hexlight (Autodesk Fusion 360 design; units mm, degrees)
Autodesk Fusion 360 part; units mm, degrees
note: some values were not read from the file. Chosen so that the rebuilt part matches the saved one: which face or edge a step refers to. Set by a fixed rule: which sketch regions a step uses.
sketch "Sketch1" plane through (0, 0, 0) normal (0, 0, 1) x (1, 0, 0)
  line L0 (86.6025, -50) -> (86.6025, 50)
  line L1 (86.6025, 50) -> (0, 100)
  line L2 (0, 100) -> (-86.6025, 50)
  line L3 (-86.6025, 50) -> (-86.6025, -50)
  line L4 (-86.6025, -50) -> (0, -100)
  line L5 (0, -100) -> (86.6025, -50)
  line L6 (0, -104.6188) -> (90.6025, -52.3094)
  line L7 (90.6025, -52.3094) -> (90.6025, 52.3094)
  line L8 (90.6025, 52.3094) -> (0, 104.6188)
  line L9 (0, 104.6188) -> (-90.6025, 52.3094)
  line L10 (-90.6025, 52.3094) -> (-90.6025, -52.3094)
  line L11 (-90.6025, -52.3094) -> (0, -104.6188)
  line L12 (0, 0) -> (0, -155)
  line L13 (0, -98.8453) -> (85.6025, -49.4226)
  line L14 (85.6025, -49.4226) -> (85.6025, 49.4226)
  line L15 (85.6025, 49.4226) -> (0, 98.8453)
  line L16 (0, 98.8453) -> (-85.6025, 49.4226)
  line L17 (-85.6025, 49.4226) -> (-85.6025, -49.4226)
  line L18 (-85.6025, -49.4226) -> (0, -98.8453)
  line L19 (0, -97.4597) -> (84.4025, -48.7298)
  line L20 (84.4025, -48.7298) -> (84.4025, 48.7298)
  line L21 (84.4025, 48.7298) -> (0, 97.4597)
  line L22 (0, 97.4597) -> (-84.4025, 48.7298)
  line L23 (-84.4025, 48.7298) -> (-84.4025, -48.7298)
  line L24 (-84.4025, -48.7298) -> (0, -97.4597)
  line L25 (-85.6025, -44.4226) -> (-84.4025, -44.4226)
  line L26 (-81.2724, -51.9226) -> (-80.6724, -50.8834)
  line L27 (-56.9017, -65.9931) -> (-56.3017, -64.9539)
  line L28 (-28.2008, -82.5635) -> (-27.6008, -81.5243)
  line L29 (-60.6318, -62.4539) -> (-61.2318, -63.4931)
  line L30 (-55.0893, -65.6539) -> (-55.6893, -66.6931)
  line L31 (-31.931, -79.0243) -> (-32.531, -80.0635)
  line L32 (-23.2707, -84.0243) -> (-23.8707, -85.0635)
  line L33 (61.1318, -62.1652) -> (61.7318, -63.2044)
  line L34 (52.4716, -67.1652) -> (53.0716, -68.2044)
  line L35 (29.3133, -80.5356) -> (29.9133, -81.5749)
  line L36 (23.7707, -83.7356) -> (24.3707, -84.7749)
  line L37 (4.3301, -96.3453) -> (3.7301, -95.3061)
  line L38 (-4.3301, -96.3453) -> (-3.7301, -95.3061)
  line L39 (84.4025, 21.8591) -> (85.6025, 21.8591)
  line L40 (84.4025, 11.8591) -> (85.6025, 11.8591)
  line L41 (84.4025, -14.8818) -> (85.6025, -14.8818)
  line L42 (84.4025, -21.2818) -> (85.6025, -21.2818)
  line L43 (85.6025, -44.4226) -> (84.4025, -44.4226)
  line L44 (81.2724, -51.9226) -> (80.6724, -50.8834)
  line L45 (23.2707, 84.0243) -> (23.8707, 85.0635)
  line L46 (31.931, 79.0243) -> (32.531, 80.0635)
  line L47 (55.0893, 65.6539) -> (55.6893, 66.6931)
  line L48 (60.6318, 62.4539) -> (61.2318, 63.4931)
  line L49 (81.2724, 51.9226) -> (80.6724, 50.8834)
  line L50 (85.6025, 44.4226) -> (84.4025, 44.4226)
  line L51 (-61.1318, 62.1652) -> (-61.7318, 63.2044)
  line L52 (-52.4716, 67.1652) -> (-53.0716, 68.2044)
  line L53 (-29.3133, 80.5356) -> (-29.9133, 81.5749)
  line L54 (-23.7707, 83.7356) -> (-24.3707, 84.7749)
  line L55 (-4.3301, 96.3453) -> (-3.7301, 95.3061)
  line L56 (4.3301, 96.3453) -> (3.7301, 95.3061)
  line L57 (-84.4025, -21.8591) -> (-85.6025, -21.8591)
  line L58 (-84.4025, -11.8591) -> (-85.6025, -11.8591)
  line L59 (-84.4025, 14.8818) -> (-85.6025, 14.8818)
  line L60 (-84.4025, 21.2818) -> (-85.6025, 21.2818)
  line L61 (-85.6025, 44.4226) -> (-84.4025, 44.4226)
  line L62 (-81.2724, 51.9226) -> (-80.6724, 50.8834)
  line L63 (-85.6025, -41.9226) -> (-84.4025, -41.9226)
  line L64 (-78.5073, -52.1334) -> (-79.1073, -53.1726)
  line L65 (-6.4952, -95.0953) -> (-5.8952, -94.0561)
  line L66 (5.8952, -94.0561) -> (6.4952, -95.0953)
  line L67 (79.1073, -53.1726) -> (78.5073, -52.1334)
  line L68 (84.4025, -41.9226) -> (85.6025, -41.9226)
  line L69 (85.6025, 41.9226) -> (84.4025, 41.9226)
  line L70 (78.5073, 52.1334) -> (79.1073, 53.1726)
  line L71 (6.4952, 95.0953) -> (5.8952, 94.0561)
  line L72 (-5.8952, 94.0561) -> (-6.4952, 95.0953)
  line L73 (-79.1073, 53.1726) -> (-78.5073, 52.1334)
  line L74 (-84.4025, 41.9226) -> (-85.6025, 41.9226)
  line L75 (-84.4025, -41.9226) -> (-83.1025, -41.9226)
  line L76 (-83.1025, -41.9226) -> (-83.1025, -44.4226)
  line L77 (-83.1025, -44.4226) -> (-84.4025, -44.4226)
  line L78 (-80.6724, -50.8834) -> (-80.0224, -49.7576)
  line L79 (-78.5073, -52.1334) -> (-77.8573, -51.0076)
  line L80 (-77.8573, -51.0076) -> (-80.0224, -49.7576)
  line L81 (-5.8952, -94.0561) -> (-5.2452, -92.9302)
  line L82 (-5.2452, -92.9302) -> (-3.0801, -94.1802)
  line L83 (-3.0801, -94.1802) -> (-3.7301, -95.3061)
  line L84 (3.7301, -95.3061) -> (3.0801, -94.1802)
  line L85 (5.2452, -92.9302) -> (3.0801, -94.1802)
  line L86 (5.8952, -94.0561) -> (5.2452, -92.9302)
  line L87 (78.5073, -52.1334) -> (77.8573, -51.0076)
  line L88 (77.8573, -51.0076) -> (80.0224, -49.7576)
  line L89 (80.0224, -49.7576) -> (80.6724, -50.8834)
  line L90 (84.4025, -44.4226) -> (83.1025, -44.4226)
  line L91 (83.1025, -41.9226) -> (83.1025, -44.4226)
  line L92 (84.4025, -41.9226) -> (83.1025, -41.9226)
  line L93 (84.4025, 41.9226) -> (83.1025, 41.9226)
  line L94 (83.1025, 41.9226) -> (83.1025, 44.4226)
  line L95 (83.1025, 44.4226) -> (84.4025, 44.4226)
  line L96 (80.6724, 50.8834) -> (80.0224, 49.7576)
  line L97 (77.8573, 51.0076) -> (80.0224, 49.7576)
  line L98 (78.5073, 52.1334) -> (77.8573, 51.0076)
  line L99 (5.8952, 94.0561) -> (5.2452, 92.9302)
  line L100 (5.2452, 92.9302) -> (3.0801, 94.1802)
  line L101 (3.0801, 94.1802) -> (3.7301, 95.3061)
  line L102 (-3.7301, 95.3061) -> (-3.0801, 94.1802)
  line L103 (-5.2452, 92.9302) -> (-3.0801, 94.1802)
  line L104 (-5.8952, 94.0561) -> (-5.2452, 92.9302)
  line L105 (-78.5073, 52.1334) -> (-77.8573, 51.0076)
  line L106 (-77.8573, 51.0076) -> (-80.0224, 49.7576)
  line L107 (-80.0224, 49.7576) -> (-80.6724, 50.8834)
  line L108 (-84.4025, 44.4226) -> (-83.1025, 44.4226)
  line L109 (-83.1025, 41.9226) -> (-83.1025, 44.4226)
  line L110 (-84.4025, 41.9226) -> (-83.1025, 41.9226)
  dimension "d1" = 100
  dimension "d2" = 4
  dimension "d7" = 1
  dimension "d8" = 1.2
  dimension "d9" = 5
  dimension "d10" = 5
  dimension "d11" = 98.8453
  dimension "d12" = 33.1409
  dimension "d13" = 66.2818
  dimension "d14" = 5
  dimension "d15" = 5
  dimension "d16" = 1.4
  dimension "d17" = 5
  dimension "d19" = 360
  dimension "d22" = 2.5
  dimension "d23" = 2.5
  dimension "d25" = 360
  dimension "d27" = 1.3
  dimension "d29" = 1.3
  dimension "d31" = 360
  constraint coincident L12.start origin
  constraint vertical L12
  constraint coincident L4.end L12
  constraint coincident L6.start L12
  constraint coincident L12 L13.start
  constraint coincident L12 L19.start
  constraint coincident L17 L25.start
  constraint coincident L23 L25.end
  constraint perpendicular L23 L25
  constraint coincident L18 L26.start
  constraint coincident L24 L26.end
  constraint perpendicular L24 L26
  constraint coincident L18 L27.start
  constraint coincident L24 L27.end
  constraint perpendicular L24 L27
  constraint coincident L18 L28.start
  constraint coincident L24 L28.end
  constraint perpendicular L24 L28
  constraint coincident L24 L29.start
  constraint coincident L18 L29.end
  constraint perpendicular L18 L29
  constraint coincident L24 L30.start
  constraint coincident L18 L30.end
  constraint perpendicular L18 L30
  constraint coincident L24 L31.start
  constraint coincident L18 L31.end
  constraint perpendicular L18 L31
  constraint coincident L24 L32.start
  constraint coincident L18 L32.end
  constraint perpendicular L18 L32
  constraint coincident L17 L63.start
  constraint coincident L23 L63.end
  constraint perpendicular L23 L63
  constraint coincident L24 L64.start
  constraint coincident L18 L64.end
  constraint perpendicular L18 L64
  constraint perpendicular L23 L75
  constraint perpendicular L75 L76
  constraint collinear L25 L77
  constraint perpendicular L24 L78
  constraint perpendicular L24 L79
  constraint parallel L24 L80
  measures "d1" distance of L0.start L4.end
  measures "d2" distance of L5 L6
  measures "d7" distance of L5 L13
  measures "d8" distance of L13 L19
  measures "d9" distance of L17.end L25
  measures "d10" distance of L17.end L26
  measures "d11" distance of L13.start L17.end
  measures "d12" distance of L17.end L27.start
  measures "d13" distance of L17.end L28.start
  measures "d14" distance of L28 L32
  measures "d15" distance of L28.end L31.start
  measures "d16" distance of L27.start L30.end
  measures "d17" distance of L27.start L29.end
  measures "d22" distance of L25 L63
  measures "d23" distance of L26 L64
  measures "d27" distance of L63.end L75.end
  measures "d29" distance of L26.end L78.end
extrude "Extrude1" add sketch "Sketch1" against normal blind 0.8 contours L0 L1 L2 L3 L4 L5 | L6 L7 L8 L9 L10 L11 | L12 L13 L19 L37 | L19 L20 L21 L22 L23 L24 L75 L76 L77 L78 L79 L80 L81 L82 L83 L84 L85 L86 L87 L88 L89 L90 L91 L92 L93 L94 L95 L96 L97 L98 L99 L100 L101 L102 L103 L104 L105 L106 L107 L108 L109 L110 | L12 L18 L24 L38 | L19 L84 L85 L86 | L13 L19 L37 L66 | L18 L24 L38 L65 | L24 L81 L82 L83 | L13 L19 L36 L66 | L18 L24 L32 L65 | L13 L19 L35 L36 | L18 L24 L28 L32 | L13 L19 L34 L35 | L18 L24 L28 L31 | L13 L19 L33 L34 | L18 L24 L30 L31 | L13 L19 L33 L67 | L18 L24 L27 L30 | L19 L87 L88 L89 | L13 L19 L44 L67 | L18 L24 L27 L29 | L13 L14 L19 L20 L43 L44 | L18 L24 L29 L64 | L18 L24 L26 L64 | L24 L78 L79 L80 | L20 L90 L91 L92 | L14 L20 L43 L68 | L17 L18 L23 L24 L25 L26 | L14 L20 L42 L68 | L14 L20 L41 L42 | L17 L23 L25 L63 | L23 L75 L76 L77 | L14 L20 L40 L41 | L17 L23 L57 L63 | L14 L20 L39 L40 | L17 L23 L57 L58 | L14 L20 L39 L69 | L17 L23 L58 L59 | L20 L93 L94 L95 | L14 L20 L50 L69 | L17 L23 L59 L60 | L14 L15 L20 L21 L49 L50 | L17 L23 L60 L74 | L17 L23 L61 L74 | L23 L108 L109 L110 | L21 L96 L97 L98 | L15 L21 L49 L70 | L16 L17 L22 L23 L61 L62 | L15 L21 L48 L70 | L15 L21 L47 L48 | L16 L22 L62 L73 | L22 L105 L106 L107 | L15 L21 L46 L47 | L16 L22 L51 L73 | L15 L21 L45 L46 | L16 L22 L51 L52 | L15 L21 L45 L71 | L16 L22 L52 L53 | L21 L99 L100 L101 | L15 L21 L56 L71 | L16 L22 L53 L54 | L15 L16 L21 L22 L55 L56 | L16 L22 L54 L72 | L16 L22 L55 L72 | L22 L102 L103 L104
extrude "Extrude2" add sketch "Sketch1" along normal blind 12 contours L6 L7 L8 L9 L10 L11
extrude "Extrude3" add sketch "Sketch1" along normal blind 9.5 contours L19 L84 L85 L86 | L13 L19 L37 L66 | L18 L24 L38 L65 | L24 L81 L82 L83 | L13 L19 L35 L36 | L18 L24 L28 L32 | L18 L24 L28 L31 | L13 L19 L33 L34 | L18 L24 L27 L30 | L19 L87 L88 L89 | L13 L19 L44 L67 | L18 L24 L27 L29 | L18 L24 L26 L64 | L24 L78 L79 L80 | L20 L90 L91 L92 | L14 L20 L43 L68 | L14 L20 L41 L42 | L17 L23 L25 L63 | L23 L75 L76 L77 | L14 L20 L39 L40 | L17 L23 L57 L58 | L20 L93 L94 L95 | L14 L20 L50 L69 | L17 L23 L59 L60 | L17 L23 L61 L74 | L23 L108 L109 L110 | L21 L96 L97 L98 | L15 L21 L49 L70 | L15 L21 L47 L48 | L16 L22 L62 L73 | L22 L105 L106 L107 | L15 L21 L45 L46 | L16 L22 L51 L52 | L21 L99 L100 L101 | L15 L21 L56 L71 | L16 L22 L53 L54 | L16 L22 L55 L72 | L22 L102 L103 L104
ref_plane "WorkPlane1" through (-15.8013, 27.3686, 6) normal (0.5, -0.866025, 0) x (0.866025, 0.5, 0)
sketch "Sketch4" plane through (-43.3013, 75, 0) normal (0.5, -0.866025, 0) x (0.866025, 0.5, 0)
  line L0 (-50, 0) -> (50, 0)
  line L1 (50, 0) -> (50, 12)
  line L2 (50, 12) -> (-50, 12)
  line L3 (-50, 12) -> (-50, 0)
  line L4 (10, 0) -> (6, 0)
  line L5 (6, 0) -> (6, 0.5)
  line L6 (6, 0.5) -> (10, 0.5)
  line L7 (10, 0.5) -> (10, 0)
  line L8 (6, 0.5) -> (10, 0.5)
  line L9 (10, 0.5) -> (10, 3)
  line L10 (10, 3) -> (6, 3)
  line L11 (6, 3) -> (6, 0.5)
  line L12 (10, 3) -> (6, 3)
  line L13 (6, 3) -> (6, 5.12)
  line L14 (10, 5.1981) -> (10, 3)
  line L15 (6, 5.12) -> (6, 10)
  line L16 (6, 10) -> (10, 10)
  line L17 (10, 10) -> (10, 5.1981)
  line L18 (6, 7) -> (10, 7)
  line L19 (10, 10) -> (6, 10)
  line L20 (6, 10) -> (6, 12)
  line L21 (6, 12) -> (10, 12)
  line L22 (10, 12) -> (10, 10)
  line L23 (6, 6.4) -> (-7, 6.4)
  line L24 (-7, 6.4) -> (-7, 3.6)
  line L25 (-7, 3.6) -> (6, 3.6)
  line L26 (6, 3.6) -> (6, 6.4)
  line L27 (-5, 6.4) -> (-5, 3.6)
  dimension "d33" = 0.5
  dimension "d34" = 2.5
  dimension "d35" = 10
  dimension "d36" = 3
  dimension "d37" = 4
  dimension "d38" = 40
  dimension "d86" = 0.6
  dimension "d87" = 0.6
  dimension "d129" = 2
  dimension "d130" = 11
  constraint horizontal L4
  constraint vertical L5
  constraint horizontal L6
  constraint vertical L7
  constraint coincident L0 L4.start
  constraint horizontal L8
  constraint vertical L9
  constraint horizontal L10
  constraint vertical L11
  constraint coincident L6.end L9
  constraint horizontal L12
  constraint vertical L13
  constraint vertical L14
  constraint coincident L10.end L13
  constraint vertical L15
  constraint horizontal L16
  constraint vertical L17
  constraint coincident L13 L15.start
  constraint coincident L15 L18.start
  constraint coincident L17 L18.end
  constraint perpendicular L17 L18
  constraint coincident L13.end L15.start
  constraint horizontal L19
  constraint vertical L20
  constraint horizontal L21
  constraint vertical L22
  constraint coincident L2 L20.end
  constraint coincident L15.end L20
  constraint horizontal L23
  constraint vertical L24
  constraint horizontal L25
  constraint vertical L26
  constraint coincident L15 L23.start
  constraint coincident L23 L27.start
  constraint coincident L25 L27.end
  constraint perpendicular L25 L27
  measures "d33" distance of L4 L6
  measures "d34" distance of L6.end L9.end
  measures "d35" distance of L4 L16
  measures "d36" distance of L16 L18
  measures "d37" distance of L15.end L16.end
  measures "d38" distance of L0.end L14
  measures "d86" distance of L18 L23
  measures "d87" distance of L10 L25
  measures "d129" distance of L24 L27
  measures "d130" distance of L26 L27
sketch "Sketch5" plane through (0, 0, 12) normal (0, 0, 1) x (-1, 0, 0)
  line L0 (-86.6025, 50) -> (0, 100)
  line L1 (0, 100) -> (86.6025, 50)
  line L2 (86.6025, 50) -> (86.6025, -50)
  line L3 (86.6025, -50) -> (0, -100)
  line L4 (0, -100) -> (-86.6025, -50)
  line L5 (-86.6025, -50) -> (-86.6025, 50)
  line L6 (90.6025, 52.3094) -> (0, 104.6188)
  line L7 (0, 104.6188) -> (-90.6025, 52.3094)
  line L8 (-90.6025, 52.3094) -> (-90.6025, -52.3094)
  line L9 (-90.6025, -52.3094) -> (0, -104.6188)
  line L10 (0, -104.6188) -> (90.6025, -52.3094)
  line L11 (90.6025, -52.3094) -> (90.6025, 52.3094)
  line L12 (34.641, -80) -> (42.641, -80)
  line L13 (42.641, -80) -> (46.1051, -78)
  line L14 (38.1051, -78) -> (46.1051, -78)
  line L15 (38.1051, -78) -> (34.641, -80)
  point P0 (34.641, -80)
  point P1 (38.1051, -78)
  constraint coincident P0 L12.start
  constraint coincident L10 L12.end
  constraint horizontal L12
  constraint coincident L10 L13.end
  constraint coincident P1 L14.start
  constraint parallel L12 L14
sketch "Sketch6" plane through (0, 0, 12) normal (0, 0, 1) x (1, 0, 0)
ref_plane "WorkPlane2" through (0, 0, 0) normal (0, 0, 1) x (1, 0, 0)
sketch "Sketch7" plane through (-45.3013, 78.4641, 0) normal (-0.5, 0.866025, 0) x (-0.866025, -0.5, 0)
  line L0 (-52.3094, 12) -> (-52.3094, -0.8)
  line L1 (-52.3094, -0.8) -> (52.3094, -0.8)
  line L2 (52.3094, -0.8) -> (52.3094, 12)
  line L3 (52.3094, 12) -> (-52.3094, 12)
  line L4 (-8, 10) -> (-5, 10)
  line L5 (-8, 7) -> (-5, 7)
  line L6 (-8, 3) -> (-5, 3)
  line L7 (-8, 0) -> (-5, 0)
  line L8 (5, 10) -> (7, 10)
  line L9 (7, 10) -> (7, 7)
  line L10 (7, 7) -> (5, 7)
  line L11 (5, 7) -> (5, 10)
  line L12 (7, 3) -> (5, 3)
  line L13 (5, 3) -> (5, 0)
  line L14 (5, 0) -> (7, 0)
  line L15 (7, 0) -> (7, 3)
  line L16 (5, 6.4) -> (7, 6.4)
  line L17 (7, 6.4) -> (7, 3.6)
  line L18 (7, 3.6) -> (5, 3.6)
  line L19 (5, 3.6) -> (5, 6.4)
  line L20 (-52.3094, 12) -> (52.3094, 12)
  line L21 (52.3094, 12) -> (52.3094, -0.8)
  line L22 (52.3094, -0.8) -> (-52.3094, -0.8)
  line L23 (-52.3094, -0.8) -> (-52.3094, 12)
  line L24 (0, 12) -> (-5, 12)
  line L25 (-5, 12) -> (-5, -0.8)
  line L26 (-5, -0.8) -> (0, -0.8)
  line L27 (0, -0.8) -> (0, 12)
  line L28 (0, 12) -> (5, 12)
  line L29 (5, 12) -> (5, -0.8)
  line L30 (5, -0.8) -> (0, -0.8)
  line L31 (0, -0.8) -> (0, 12)
  line L32 (-8, 12) -> (-8, -0.8)
  point P0 (0.9282, 12)
  point P1 (-3.0718, 12)
  dimension "d41" = 3
  dimension "d42" = 4
  dimension "d43" = 3
  dimension "d46" = 3
  dimension "d47" = 3
  dimension "d50" = 2
  dimension "d51" = 2
  dimension "d92" = 0.6
  dimension "d93" = 0.6
  dimension "d106" = 5
  dimension "d107" = 5
  dimension "d108" = 0.8
  dimension "d109" = 3
  constraint horizontal L8
  constraint vertical L9
  constraint horizontal L10
  constraint vertical L11
  constraint horizontal L12
  constraint vertical L13
  constraint horizontal L14
  constraint vertical L15
  constraint collinear L7 L14
  constraint collinear L5 L10
  constraint horizontal L16
  constraint vertical L17
  constraint horizontal L18
  constraint vertical L19
  constraint collinear L9 L17
  constraint collinear L11 L19
  constraint horizontal L20
  constraint vertical L21
  constraint horizontal L22
  constraint vertical L23
  constraint coincident L1.end L2.start
  constraint coincident L0.start L3.end
  constraint horizontal L24
  constraint vertical L25
  constraint horizontal L26
  constraint vertical L27
  constraint coincident L22 L25.end
  constraint midpoint L20 L24.start
  constraint horizontal L28
  constraint vertical L29
  constraint horizontal L30
  constraint vertical L31
  constraint coincident L22 L29.end
  constraint coincident L4.end L25
  constraint coincident L5.end L25
  constraint coincident L6.end L25
  constraint coincident L7.end L25
  constraint collinear L11 L29
  constraint collinear L13 L29
  constraint coincident L20 L32.start
  constraint coincident L22 L32.end
  constraint perpendicular L22 L32
  constraint coincident L4.start L32
  constraint coincident L5.start L32
  constraint coincident L6.start L32
  constraint coincident L7.start L32
  measures "d41" distance of L6 L7
  measures "d42" distance of L5 L6
  measures "d43" distance of L4 L5
  measures "d46" distance of L8.start L10.end
  measures "d47" distance of L12.end L13.end
  measures "d50" distance of L12.start L12.end
  measures "d51" distance of L8.start L8.end
  measures "d92" distance of L10 L16
  measures "d93" distance of L12 L18
  measures "d106" distance of L27 L29
  measures "d107" distance of L25 L31
  measures "d108" distance of L14 L22
  measures "d109" distance of L25 L32
sketch "Sketch15" plane through (-42.8731, 79.866, 5) normal (-0.5, 0.866025, 0) x (0.866025, 0.5, 0)
  line L0 (-7.8038, -2) -> (-9.8038, -2)
  line L1 (-9.8038, -2) -> (-9.8038, 2)
  line L2 (-9.8038, 2) -> (-7.8038, 2)
  line L3 (-7.8038, 2) -> (-7.8038, -2)
  line L4 (5.1962, -2) -> (2.1962, -2)
  line L5 (5.1962, 2) -> (2.1962, 2)
  line L6 (-7.8038, -1.4) -> (-9.8038, -1.4)
  line L7 (-9.8038, -1.4) -> (-9.8038, 1.4)
  line L8 (-9.8038, 1.4) -> (-7.8038, 1.4)
  line L9 (-7.8038, 1.4) -> (-7.8038, -1.4)
  line L10 (-7.8038, 1.4) -> (-7.8038, -1.4)
  dimension "d84" = 0.6
  dimension "d85" = 0.6
  dimension "d110" = 2
  constraint horizontal L0
  constraint vertical L1
  constraint horizontal L2
  constraint vertical L3
  constraint collinear L0 L4
  constraint collinear L2 L5
  constraint horizontal L6
  constraint vertical L7
  constraint horizontal L8
  constraint vertical L9
  constraint coincident L1 L7.end
  constraint coincident L3 L6.start
  constraint coincident L0.start L3.end
  constraint collinear L9 L10
  measures "d84" distance of L0 L6
  measures "d85" distance of L2 L8
  measures "d110" distance of L0.end L0.start
loft "Loft5" cut profiles "Sketch4", "Sketch15" section 1 contours L23 L24 L25 L27 section 2 contours L1 L3 L6 L7 L8 L9 L10
loft "Loft1" cut profiles "Sketch4", "Sketch7" section 1 contours L15 L16 L17 L18 L19 section 2 contours L4 L5 L25 L32
loft "Loft2" cut profiles "Sketch4", "Sketch7" section 1 contours L0 L4 L5 L6 L7 L8 | L6 L8 L9 L10 L11 L12 section 2 contours L6 L7 L25 L32
pattern_circular "C-Pattern1" count 6 over 360 about axis through (0, 0, 1.75) along (0, 0, 1) of 7 faces at (-35.885, 80.8214, 9) (-36.9229, 79.4524, 10) (-40.0158, 79.9761, 1) (-37.1291, 81.6427, 2) (-36.9229, 79.4524, 7) (-39.0605, 78.988, 9) (-36.9229, 79.4524, 3)
ref_plane "WorkPlane3" through (-51.0395, 68.6848, 4.75) normal (-0.866025, -0.5, 0) x (0.5, -0.866025, 0)
sketch "Sketch10" plane through (-51.0895, 68.7714, 4.75) normal (-0.866025, -0.5, 0) x (0.5, -0.866025, 0)
  line L0 (-5.5, 5.25) -> (-4.5, 5.25)
  line L1 (-4.5, 5.25) -> (-4.5, 2.25)
  line L2 (-4.5, 2.25) -> (-5.5, 2.25)
  line L3 (-5.5, 2.25) -> (-5.5, 5.25)
  line L4 (-5.5, -1.75) -> (-4.5, -1.75)
  line L5 (-4.5, -1.75) -> (-4.5, -4.75)
  line L6 (-4.5, -4.75) -> (-5.5, -4.75)
  line L7 (-5.5, -4.75) -> (-5.5, -1.75)
  line L8 (-4.5, 1.65) -> (-5.5, 1.65)
  line L9 (-5.5, 1.65) -> (-5.5, -1.15)
  line L10 (-5.5, -1.15) -> (-4.5, -1.15)
  line L11 (-4.5, -1.15) -> (-4.5, 1.65)
  line L12 (-5.5, -5.55) -> (-5.5, 7.2767)
  point P0 (-5.5, -5.55)
  dimension "d59" = 3
  dimension "d60" = 3
  dimension "d61" = 0.8
  dimension "d62" = 4
  dimension "d63" = 1
  dimension "d64" = 1
  dimension "d90" = 0.6
  dimension "d91" = 0.6
  constraint horizontal L0
  constraint vertical L1
  constraint horizontal L2
  constraint vertical L3
  constraint horizontal L4
  constraint vertical L5
  constraint horizontal L6
  constraint vertical L7
  constraint collinear L1 L5
  constraint horizontal L8
  constraint vertical L9
  constraint horizontal L10
  constraint vertical L11
  constraint collinear L5 L11
  constraint collinear L7 L9
  constraint coincident P0 L12.start
  constraint vertical L12
  constraint collinear L7 L12
  measures "d59" distance of L4.start L6.end
  measures "d60" distance of L0.start L2.end
  measures "d61" distance of L6 P0
  measures "d62" distance of L2 L4
  measures "d63" distance of L4.start L4.end
  measures "d64" distance of L1.end L2.end
  measures "d90" distance of L4 L10
  measures "d91" distance of L2 L8
loft "Loft6" [suppressed]
pattern_circular "C-Pattern5" [suppressed]
loft "Loft3" cut profiles "Sketch10", "Sketch7" section 1 contours L0 L1 L2 L3 L12 section 2 contours L8 L9 L10 L11 L29
loft "Loft4" cut profiles "Sketch10", "Sketch7" section 1 contours L4 L5 L6 L7 L12 section 2 contours L12 L13 L14 L15 L29
sketch "Sketch11" plane through (0, 0, 0) normal (0, 0, 1) x (-1, 0, 0)
  line L0 (0, -100) -> (34.641, -80)
  line L1 (38.3731, -82.4641) -> (40.9711, -80.9641)
  line L2 (86.6025, -50) -> (86.6025, -10)
  line L3 (86.6025, 50) -> (51.9615, 70)
  line L4 (0, 100) -> (-34.641, 80)
  line L5 (-86.6025, 50) -> (-86.6025, 10)
  line L6 (-48.4974, -72) -> (0, -100)
  line L7 (84.4025, -21.2818) -> (84.4025, -14.8818)
  line L8 (84.4025, -14.8818) -> (85.6025, -14.8818)
  line L9 (85.6025, -14.8818) -> (85.6025, -21.2818)
  line L10 (85.6025, -21.2818) -> (84.4025, -21.2818)
  line L11 (-4.3301, 96.3453) -> (-3.0801, 94.1802)
  line L12 (-3.0801, 94.1802) -> (-5.2452, 92.9302)
  line L13 (-5.2452, 92.9302) -> (-6.4952, 95.0953)
  line L14 (-6.4952, 95.0953) -> (-4.3301, 96.3453)
  line L15 (-84.4025, -21.8591) -> (-85.6025, -21.8591)
  line L16 (-85.6025, -21.8591) -> (-85.6025, -11.8591)
  line L17 (-85.6025, -11.8591) -> (-84.4025, -11.8591)
  line L18 (-84.4025, -11.8591) -> (-84.4025, -21.8591)
  line L19 (-23.2707, -84.0243) -> (-23.8707, -85.0635)
  line L20 (-23.8707, -85.0635) -> (-32.531, -80.0635)
  line L21 (-32.531, -80.0635) -> (-31.931, -79.0243)
  line L22 (-31.931, -79.0243) -> (-23.2707, -84.0243)
  line L23 (61.1318, -62.1652) -> (61.7318, -63.2044)
  line L24 (61.7318, -63.2044) -> (53.0716, -68.2044)
  line L25 (53.0716, -68.2044) -> (52.4716, -67.1652)
  line L26 (52.4716, -67.1652) -> (61.1318, -62.1652)
  line L27 (84.4025, 21.8591) -> (85.6025, 21.8591)
  line L28 (85.6025, 21.8591) -> (85.6025, 11.8591)
  line L29 (85.6025, 11.8591) -> (84.4025, 11.8591)
  line L30 (84.4025, 11.8591) -> (84.4025, 21.8591)
  line L31 (31.931, 79.0243) -> (23.2707, 84.0243)
  line L32 (23.2707, 84.0243) -> (23.8707, 85.0635)
  line L33 (23.8707, 85.0635) -> (32.531, 80.0635)
  line L34 (32.531, 80.0635) -> (31.931, 79.0243)
  line L35 (6.4952, 95.0953) -> (5.2452, 92.9302)
  line L36 (5.2452, 92.9302) -> (3.0801, 94.1802)
  line L37 (3.0801, 94.1802) -> (4.3301, 96.3453)
  line L38 (4.3301, 96.3453) -> (6.4952, 95.0953)
  line L39 (85.6025, 41.9226) -> (83.1025, 41.9226)
  line L40 (83.1025, 41.9226) -> (83.1025, 44.4226)
  line L41 (83.1025, 44.4226) -> (85.6025, 44.4226)
  line L42 (85.6025, 44.4226) -> (85.6025, 41.9226)
  line L43 (79.1073, -53.1726) -> (77.8573, -51.0076)
  line L44 (77.8573, -51.0076) -> (80.0224, -49.7576)
  line L45 (80.0224, -49.7576) -> (81.2724, -51.9226)
  line L46 (81.2724, -51.9226) -> (79.1073, -53.1726)
  line L47 (-6.4952, -95.0953) -> (-5.2452, -92.9302)
  line L48 (-5.2452, -92.9302) -> (-3.0801, -94.1802)
  line L49 (-3.0801, -94.1802) -> (-4.3301, -96.3453)
  line L50 (-4.3301, -96.3453) -> (-6.4952, -95.0953)
  line L51 (-85.6025, -41.9226) -> (-83.1025, -41.9226)
  line L52 (-83.1025, -41.9226) -> (-83.1025, -44.4226)
  line L53 (-83.1025, -44.4226) -> (-85.6025, -44.4226)
  line L54 (-85.6025, -44.4226) -> (-85.6025, -41.9226)
  line L55 (-61.1318, 62.1652) -> (-61.7318, 63.2044)
  line L56 (-61.7318, 63.2044) -> (-53.0716, 68.2044)
  line L57 (-53.0716, 68.2044) -> (-52.4716, 67.1652)
  line L58 (-52.4716, 67.1652) -> (-61.1318, 62.1652)
  line L59 (29.3133, -80.5356) -> (29.9133, -81.5749)
  line L60 (29.9133, -81.5749) -> (24.3707, -84.7749)
  line L61 (24.3707, -84.7749) -> (23.7707, -83.7356)
  line L62 (23.7707, -83.7356) -> (29.3133, -80.5356)
  line L63 (79.1073, 53.1726) -> (81.2724, 51.9226)
  line L64 (81.2724, 51.9226) -> (80.0224, 49.7576)
  line L65 (80.0224, 49.7576) -> (77.8573, 51.0076)
  line L66 (77.8573, 51.0076) -> (79.1073, 53.1726)
  line L67 (85.6025, -44.4226) -> (83.1025, -44.4226)
  line L68 (83.1025, -44.4226) -> (83.1025, -41.9226)
  line L69 (83.1025, -41.9226) -> (85.6025, -41.9226)
  line L70 (85.6025, -41.9226) -> (85.6025, -44.4226)
  line L71 (4.3301, -96.3453) -> (3.0801, -94.1802)
  line L72 (3.0801, -94.1802) -> (5.2452, -92.9302)
  line L73 (5.2452, -92.9302) -> (6.4952, -95.0953)
  line L74 (6.4952, -95.0953) -> (4.3301, -96.3453)
  line L75 (-81.2724, -51.9226) -> (-80.0224, -49.7576)
  line L76 (-80.0224, -49.7576) -> (-77.8573, -51.0076)
  line L77 (-77.8573, -51.0076) -> (-79.1073, -53.1726)
  line L78 (-79.1073, -53.1726) -> (-81.2724, -51.9226)
  line L79 (-85.6025, 44.4226) -> (-83.1025, 44.4226)
  line L80 (-83.1025, 44.4226) -> (-83.1025, 41.9226)
  line L81 (-83.1025, 41.9226) -> (-85.6025, 41.9226)
  line L82 (-85.6025, 41.9226) -> (-85.6025, 44.4226)
  line L83 (-79.1073, 53.1726) -> (-77.8573, 51.0076)
  line L84 (-77.8573, 51.0076) -> (-80.0224, 49.7576)
  line L85 (-80.0224, 49.7576) -> (-81.2724, 51.9226)
  line L86 (-81.2724, 51.9226) -> (-79.1073, 53.1726)
  line L87 (55.6893, 66.6931) -> (61.2318, 63.4931)
  line L88 (61.2318, 63.4931) -> (60.6318, 62.4539)
  line L89 (60.6318, 62.4539) -> (55.0893, 65.6539)
  line L90 (55.0893, 65.6539) -> (55.6893, 66.6931)
  line L91 (-29.9133, 81.5749) -> (-24.3707, 84.7749)
  line L92 (-24.3707, 84.7749) -> (-23.7707, 83.7356)
  line L93 (-23.7707, 83.7356) -> (-29.3133, 80.5356)
  line L94 (-29.3133, 80.5356) -> (-29.9133, 81.5749)
  line L95 (-85.6025, 14.8818) -> (-85.6025, 21.2818)
  line L96 (-85.6025, 21.2818) -> (-84.4025, 21.2818)
  line L97 (-84.4025, 21.2818) -> (-84.4025, 14.8818)
  line L98 (-84.4025, 14.8818) -> (-85.6025, 14.8818)
  line L99 (-55.6893, -66.6931) -> (-61.2318, -63.4931)
  line L100 (-61.2318, -63.4931) -> (-60.6318, -62.4539)
  line L101 (-60.6318, -62.4539) -> (-55.0893, -65.6539)
  line L102 (-55.0893, -65.6539) -> (-55.6893, -66.6931)
  line L103 (86.6025, 7) -> (-0.415, 7)
  line L104 (-0.415, 7) -> (-0.415, 5)
  line L105 (-0.415, 5) -> (86.6025, 5)
  line L106 (86.6025, 5) -> (86.6025, 7)
  line L107 (34.641, -80) -> (38.3731, -82.4641)
  line L108 (40.9711, -80.9641) -> (38.1051, -78)
  line L109 (38.1051, -78) -> (86.6025, -50)
  line L110 (-51.9615, -70) -> (-52.2295, -74.4641)
  line L111 (-52.2295, -74.4641) -> (-49.6314, -75.9641)
  line L112 (-49.6314, -75.9641) -> (-48.4974, -72)
  line L113 (86.6025, -10) -> (90.6025, -8)
  line L114 (90.6025, -8) -> (90.6025, -5)
  line L115 (90.6025, -5) -> (86.6025, -6)
  line L116 (86.6025, -6) -> (86.6025, 50)
  line L117 (51.9615, 70) -> (52.2295, 74.4641)
  line L118 (52.2295, 74.4641) -> (49.6314, 75.9641)
  line L119 (49.6314, 75.9641) -> (48.4974, 72)
  line L120 (48.4974, 72) -> (0, 100)
  line L121 (-34.641, 80) -> (-38.3731, 82.4641)
  line L122 (-38.3731, 82.4641) -> (-40.9711, 80.9641)
  line L123 (-40.9711, 80.9641) -> (-38.1051, 78)
  line L124 (-38.1051, 78) -> (-86.6025, 50)
  line L125 (-86.6025, 10) -> (-90.6025, 8)
  line L126 (-90.6025, 8) -> (-90.6025, 5)
  line L127 (-90.6025, 5) -> (-86.6025, 6)
  line L128 (-86.6025, 6) -> (-86.6025, -50)
  line L129 (-86.6025, -50) -> (-51.9615, -70)
  dimension "d66" = 2
  constraint horizontal L103
  constraint vertical L104
  constraint horizontal L105
  constraint vertical L106
  constraint coincident L103.end L104.start
  measures "d66" distance of L103.start L105.end
extrude "Extrude4" cut sketch "Sketch11" against normal blind 0.4 contours L103 L104 L105 L106 L116
pattern_circular "C-Pattern2" count 6 over 360 about axis through (0, 0, 1.75) along (0, 0, 1) of "Extrude4"
pattern_circular "C-Pattern3" count 6 over 360 about axis through (0, 0, 1.75) along (0, 0, 1) of 8 faces at (-53.0742, 73.4953, 10) (-53.0742, 73.4953, 3) (-53.0742, 73.4953, 7) (-53.5062, 72.9572, 9) (-52.1035, 73.767, 9) (-53.0742, 73.4953, 0) (-53.6728, 73.2459, 1) (-50.8674, 74.8656, 1)
sketch "Sketch12" plane through (0, 0, 0) normal (0, 0, 1) x (-1, 0, 0)
  line L0 (0.415, -7) -> (-86.6025, -7)
  circle A0 centre (0, 0) radius 7.5
  line L1 (49.3634, -71.5) -> (86.6025, -50)
  line L2 (86.6025, -50) -> (86.6025, -10)
  line L3 (86.6025, 50) -> (51.9615, 70)
  line L4 (0, 100) -> (-34.641, 80)
  line L5 (-86.6025, 50) -> (-86.6025, 10)
  line L6 (-86.6025, -50) -> (-51.9615, -70)
  line L7 (38.3731, -82.4641) -> (40.9711, -80.9641)
  line L8 (-55.6893, -66.6931) -> (-61.2318, -63.4931)
  line L9 (-61.2318, -63.4931) -> (-60.6318, -62.4539)
  line L10 (-60.6318, -62.4539) -> (-55.0893, -65.6539)
  line L11 (-55.0893, -65.6539) -> (-55.6893, -66.6931)
  line L12 (-29.9133, 81.5749) -> (-24.3707, 84.7749)
  line L13 (-24.3707, 84.7749) -> (-23.7707, 83.7356)
  line L14 (-23.7707, 83.7356) -> (-29.3133, 80.5356)
  line L15 (-29.3133, 80.5356) -> (-29.9133, 81.5749)
  line L16 (-4.3301, 96.3453) -> (-3.0801, 94.1802)
  line L17 (-3.0801, 94.1802) -> (-5.2452, 92.9302)
  line L18 (-5.2452, 92.9302) -> (-6.4952, 95.0953)
  line L19 (-6.4952, 95.0953) -> (-4.3301, 96.3453)
  line L20 (-84.4025, -21.8591) -> (-85.6025, -21.8591)
  line L21 (-85.6025, -21.8591) -> (-85.6025, -11.8591)
  line L22 (-85.6025, -11.8591) -> (-84.4025, -11.8591)
  line L23 (-84.4025, -11.8591) -> (-84.4025, -21.8591)
  line L24 (-23.2707, -84.0243) -> (-23.8707, -85.0635)
  line L25 (-23.8707, -85.0635) -> (-32.531, -80.0635)
  line L26 (-32.531, -80.0635) -> (-31.931, -79.0243)
  line L27 (-31.931, -79.0243) -> (-23.2707, -84.0243)
  line L28 (61.1318, -62.1652) -> (61.7318, -63.2044)
  line L29 (61.7318, -63.2044) -> (53.0716, -68.2044)
  line L30 (53.0716, -68.2044) -> (52.4716, -67.1652)
  line L31 (52.4716, -67.1652) -> (61.1318, -62.1652)
  line L32 (84.4025, 21.8591) -> (85.6025, 21.8591)
  line L33 (85.6025, 21.8591) -> (85.6025, 11.8591)
  line L34 (85.6025, 11.8591) -> (84.4025, 11.8591)
  line L35 (84.4025, 11.8591) -> (84.4025, 21.8591)
  line L36 (31.931, 79.0243) -> (23.2707, 84.0243)
  line L37 (23.2707, 84.0243) -> (23.8707, 85.0635)
  line L38 (23.8707, 85.0635) -> (32.531, 80.0635)
  line L39 (32.531, 80.0635) -> (31.931, 79.0243)
  line L40 (6.4952, 95.0953) -> (5.2452, 92.9302)
  line L41 (5.2452, 92.9302) -> (3.0801, 94.1802)
  line L42 (3.0801, 94.1802) -> (4.3301, 96.3453)
  line L43 (4.3301, 96.3453) -> (6.4952, 95.0953)
  line L44 (85.6025, 41.9226) -> (83.1025, 41.9226)
  line L45 (83.1025, 41.9226) -> (83.1025, 44.4226)
  line L46 (83.1025, 44.4226) -> (85.6025, 44.4226)
  line L47 (85.6025, 44.4226) -> (85.6025, 41.9226)
  line L48 (79.1073, -53.1726) -> (77.8573, -51.0076)
  line L49 (77.8573, -51.0076) -> (80.0224, -49.7576)
  line L50 (80.0224, -49.7576) -> (81.2724, -51.9226)
  line L51 (81.2724, -51.9226) -> (79.1073, -53.1726)
  line L52 (-6.4952, -95.0953) -> (-5.2452, -92.9302)
  line L53 (-5.2452, -92.9302) -> (-3.0801, -94.1802)
  line L54 (-3.0801, -94.1802) -> (-4.3301, -96.3453)
  line L55 (-4.3301, -96.3453) -> (-6.4952, -95.0953)
  line L56 (-85.6025, -41.9226) -> (-83.1025, -41.9226)
  line L57 (-83.1025, -41.9226) -> (-83.1025, -44.4226)
  line L58 (-83.1025, -44.4226) -> (-85.6025, -44.4226)
  line L59 (-85.6025, -44.4226) -> (-85.6025, -41.9226)
  line L60 (-61.1318, 62.1652) -> (-61.7318, 63.2044)
  line L61 (-61.7318, 63.2044) -> (-53.0716, 68.2044)
  line L62 (-53.0716, 68.2044) -> (-52.4716, 67.1652)
  line L63 (-52.4716, 67.1652) -> (-61.1318, 62.1652)
  line L64 (29.3133, -80.5356) -> (29.9133, -81.5749)
  line L65 (29.9133, -81.5749) -> (24.3707, -84.7749)
  line L66 (24.3707, -84.7749) -> (23.7707, -83.7356)
  line L67 (23.7707, -83.7356) -> (29.3133, -80.5356)
  line L68 (79.1073, 53.1726) -> (81.2724, 51.9226)
  line L69 (81.2724, 51.9226) -> (80.0224, 49.7576)
  line L70 (80.0224, 49.7576) -> (77.8573, 51.0076)
  line L71 (77.8573, 51.0076) -> (79.1073, 53.1726)
  line L72 (85.6025, -44.4226) -> (83.1025, -44.4226)
  line L73 (83.1025, -44.4226) -> (83.1025, -41.9226)
  line L74 (83.1025, -41.9226) -> (85.6025, -41.9226)
  line L75 (85.6025, -41.9226) -> (85.6025, -44.4226)
  line L76 (4.3301, -96.3453) -> (3.0801, -94.1802)
  line L77 (3.0801, -94.1802) -> (5.2452, -92.9302)
  line L78 (5.2452, -92.9302) -> (6.4952, -95.0953)
  line L79 (6.4952, -95.0953) -> (4.3301, -96.3453)
  line L80 (-81.2724, -51.9226) -> (-80.0224, -49.7576)
  line L81 (-80.0224, -49.7576) -> (-77.8573, -51.0076)
  line L82 (-77.8573, -51.0076) -> (-79.1073, -53.1726)
  line L83 (-79.1073, -53.1726) -> (-81.2724, -51.9226)
  line L84 (-85.6025, 44.4226) -> (-83.1025, 44.4226)
  line L85 (-83.1025, 44.4226) -> (-83.1025, 41.9226)
  line L86 (-83.1025, 41.9226) -> (-85.6025, 41.9226)
  line L87 (-85.6025, 41.9226) -> (-85.6025, 44.4226)
  line L88 (-79.1073, 53.1726) -> (-77.8573, 51.0076)
  line L89 (-77.8573, 51.0076) -> (-80.0224, 49.7576)
  line L90 (-80.0224, 49.7576) -> (-81.2724, 51.9226)
  line L91 (-81.2724, 51.9226) -> (-79.1073, 53.1726)
  line L92 (85.6025, -14.8818) -> (85.6025, -21.2818)
  line L93 (85.6025, -21.2818) -> (84.4025, -21.2818)
  line L94 (84.4025, -21.2818) -> (84.4025, -14.8818)
  line L95 (84.4025, -14.8818) -> (85.6025, -14.8818)
  line L96 (55.6893, 66.6931) -> (61.2318, 63.4931)
  line L97 (61.2318, 63.4931) -> (60.6318, 62.4539)
  line L98 (60.6318, 62.4539) -> (55.0893, 65.6539)
  line L99 (55.0893, 65.6539) -> (55.6893, 66.6931)
  line L100 (-85.6025, 14.8818) -> (-85.6025, 21.2818)
  line L101 (-85.6025, 21.2818) -> (-84.4025, 21.2818)
  line L102 (-84.4025, 21.2818) -> (-84.4025, 14.8818)
  line L103 (-84.4025, 14.8818) -> (-85.6025, 14.8818)
  line L104 (34.641, -80) -> (38.3731, -82.4641)
  line L105 (40.9711, -80.9641) -> (38.1051, -78)
  line L106 (86.6025, -10) -> (90.6025, -8)
  line L107 (90.6025, -8) -> (90.6025, -5)
  line L108 (90.6025, -5) -> (86.6025, -6)
  line L109 (86.6025, -6) -> (86.6025, 5)
  line L110 (86.6025, 7) -> (86.6025, 50)
  line L111 (51.9615, 70) -> (52.2295, 74.4641)
  line L112 (52.2295, 74.4641) -> (49.6314, 75.9641)
  line L113 (49.6314, 75.9641) -> (48.4974, 72)
  line L114 (48.4974, 72) -> (38.9711, 77.5)
  line L115 (37.2391, 78.5) -> (0, 100)
  line L116 (-34.641, 80) -> (-38.3731, 82.4641)
  line L117 (-38.3731, 82.4641) -> (-40.9711, 80.9641)
  line L118 (-40.9711, 80.9641) -> (-38.1051, 78)
  line L119 (-38.1051, 78) -> (-47.6314, 72.5)
  line L120 (-49.3634, 71.5) -> (-86.6025, 50)
  line L121 (-86.6025, 10) -> (-90.6025, 8)
  line L122 (-90.6025, 8) -> (-90.6025, 5)
  line L123 (-90.6025, 5) -> (-86.6025, 6)
  line L124 (-86.6025, 6) -> (-86.6025, -5)
  line L125 (-86.6025, -7) -> (-86.6025, -50)
  line L126 (-51.9615, -70) -> (-52.2295, -74.4641)
  line L127 (-52.2295, -74.4641) -> (-49.6314, -75.9641)
  line L128 (-49.6314, -75.9641) -> (-48.4974, -72)
  line L129 (-48.4974, -72) -> (-38.9711, -77.5)
  line L130 (-37.2391, -78.5) -> (0, -100)
  line L131 (0, -100) -> (34.641, -80)
  line L132 (38.1051, -78) -> (47.6314, -72.5)
  dimension "d132" = 15
  constraint coincident A0.centre origin
  measures "d132" diameter of A0
sketch "Sketch16" plane through (-43.3013, 75, 0) normal (0.5, -0.866025, 0) x (0.866025, 0.5, 0)
  line L0 (-7, 0) -> (-7, -0.4)
  line L1 (-5, -0.4) -> (-5, 0)
  line L2 (-5, 0) -> (6, 0)
  line L3 (6, 3) -> (10, 3)
  line L4 (50, 0) -> (50, 12)
  line L5 (50, 12) -> (-50, 12)
  line L6 (-50, 12) -> (-50, 0)
  line L7 (10, 7) -> (6, 7)
  line L8 (6, 10) -> (10, 10)
  line L9 (-7, -0.4) -> (-5, -0.4)
  line L10 (-7, 6.4) -> (-5, 6.4)
  line L11 (-5, 6.4) -> (-5, 3.6)
  line L12 (-5, 3.6) -> (-7, 3.6)
  line L13 (6, 0) -> (6, 3)
  line L14 (10, 3) -> (10, 0)
  line L15 (6, 7) -> (6, 10)
  line L16 (10, 10) -> (10, 7)
  line L17 (-7, 3.6) -> (-7, 6.4)
  line L18 (10, 0) -> (50, 0)
  line L19 (-50, 0) -> (-7, 0)
extrude "Extrude5" cut sketch "Sketch12" against normal blind 0.4 contours A0
sketch "Sketch13" plane through (43.3013, 75, 0) normal (-0.5, -0.866025, 0) x (0.866025, -0.5, 0)
  line L0 (-7, 0) -> (-7, -0.4)
  line L1 (-7, -0.4) -> (-5, -0.4)
  line L2 (-5, -0.4) -> (-5, 0)
  line L3 (-5, 0) -> (6, 0)
  line L4 (50, 0) -> (50, 12)
  line L5 (50, 12) -> (-50, 12)
  line L6 (-50, 12) -> (-50, 0)
  line L7 (-5, -0.4) -> (-7, -0.4)
  line L8 (-7, -0.4) -> (-7, 6.4)
  line L9 (-7, 6.4) -> (-5, 6.4)
  line L10 (-5, 6.4) -> (-5, -0.4)
  line L11 (6, 0) -> (6, 3)
  line L12 (6, 3) -> (10, 3)
  line L13 (10, 3) -> (10, 0)
  line L14 (10, 0) -> (50, 0)
  line L15 (-50, 0) -> (-7, 0)
  line L16 (10, 7) -> (6, 7)
  line L17 (6, 7) -> (6, 10)
  line L18 (6, 10) -> (10, 10)
  line L19 (10, 10) -> (10, 7)
  constraint horizontal L7
  constraint vertical L8
  constraint horizontal L9
  constraint vertical L10
  constraint coincident L1.end L2.start
  constraint coincident L0.end L1.start
extrude "Extrude6" cut sketch "Sketch13" against normal blind 0.5 contours L0 L1 L2 L7 L8 L9 L10
pattern_circular "C-Pattern4" count 6 over 360 about axis through (0, 0, 1.75) along (0, 0, 1) of "Extrude6"
sketch "Sketch18" plane through (0, 0, 12) normal (0, 0, 1) x (-1, 0, 0)
  line L0 (-86.6025, 50) -> (0, 100)
  line L1 (0, 100) -> (86.6025, 50)
  line L2 (86.6025, 50) -> (86.6025, -50)
  line L3 (86.6025, -50) -> (0, -100)
  line L4 (0, -100) -> (-86.6025, -50)
  line L5 (-86.6025, -50) -> (-86.6025, 50)
  line L6 (90.6025, 52.3094) -> (0, 104.6188)
  line L7 (0, 104.6188) -> (-90.6025, 52.3094)
  line L8 (-90.6025, 52.3094) -> (-90.6025, -52.3094)
  line L9 (-90.6025, -52.3094) -> (0, -104.6188)
  line L10 (0, -104.6188) -> (90.6025, -52.3094)
  line L11 (90.6025, -52.3094) -> (90.6025, 52.3094)
  line L12 (86.6025, -50) -> (-86.6025, 50)
  constraint coincident L2.end L3.start
  constraint coincident L0.start L5.end
ref_plane "WorkPlane4" through (0, 0, 12) normal (0.5, 0.866025, 0) x (0.866025, -0.5, 0)
sketch "Sketch21" plane through (0, 0, 12) normal (0, 0, 1) x (-1, 0, 0)
  line L0 (-86.6025, 50) -> (0, 100)
  line L1 (0, 100) -> (86.6025, 50)
  line L2 (86.6025, 50) -> (86.6025, -50)
  line L3 (86.6025, -50) -> (0, -100)
  line L4 (0, -100) -> (-86.6025, -50)
  line L5 (-86.6025, -50) -> (-86.6025, 50)
  line L6 (90.6025, 52.3094) -> (0, 104.6188)
  line L7 (0, 104.6188) -> (-90.6025, 52.3094)
  line L8 (-90.6025, 52.3094) -> (-90.6025, -52.3094)
  line L9 (-90.6025, -52.3094) -> (0, -104.6188)
  line L10 (0, -104.6188) -> (90.6025, -52.3094)
  line L11 (90.6025, -52.3094) -> (90.6025, 52.3094)
  line L12 (-86.6025, 44.5) -> (-88.8025, 44.5)
  line L13 (-88.8025, 44.5) -> (-88.8025, 32.5)
  line L14 (-88.8025, 32.5) -> (-86.6025, 32.5)
  line L15 (-86.6025, 32.5) -> (-86.6025, 44.5)
  line L16 (0, 0) -> (-110, 0)
  line L17 (-88.8025, -44.5) -> (-88.8025, -32.5)
  line L18 (-88.8025, -32.5) -> (-86.6025, -32.5)
  line L19 (-86.6025, -44.5) -> (-88.8025, -44.5)
  line L20 (-86.6025, -32.5) -> (-86.6025, -44.5)
  dimension "d112" = 2.2
  dimension "d113" = 12
  dimension "d114" = 5.5
  dimension "d119" = 110
  constraint horizontal L12
  constraint vertical L13
  constraint horizontal L14
  constraint vertical L15
  constraint coincident L5 L12.start
  constraint coincident L16.start origin
  constraint horizontal L16
  constraint symmetric L12.start L16 L19.start
  constraint symmetric L12.end L16 L17.start
  constraint symmetric L13.end L16 L17.end
  constraint symmetric L14.end L16 L18.end
  measures "d112" distance of L13.end L14.end
  measures "d113" distance of L12.end L13.end
  measures "d114" distance of L0.start L12
  measures "d119" distance of L16.start L16.end
extrude "Extrude8" cut sketch "Sketch21" against normal up to surface (12 mm away) contours L5 L12 L13 L14 L15 | L5 L17 L18 L19 L20
pattern_circular "C-Pattern6" count 6 over 360 about axis through (0, 0, 1.75) along (0, 0, 1) of "Extrude8"
sketch "Sketch22" plane through (0, 0, 0) normal (0, 0, 1) x (-1, 0, 0)
  line L0 (4.3301, -96.3453) -> (3.0801, -94.1802)
  line L1 (3.0801, -94.1802) -> (5.2452, -92.9302)
  line L2 (5.2452, -92.9302) -> (6.4952, -95.0953)
  line L3 (6.4952, -95.0953) -> (4.3301, -96.3453)
  line L4 (29.3133, -80.5356) -> (29.9133, -81.5749)
  line L5 (29.9133, -81.5749) -> (24.3707, -84.7749)
  line L6 (24.3707, -84.7749) -> (23.7707, -83.7356)
  line L7 (23.7707, -83.7356) -> (29.3133, -80.5356)
  line L8 (-23.2707, -84.0243) -> (-23.8707, -85.0635)
  line L9 (-23.8707, -85.0635) -> (-32.531, -80.0635)
  line L10 (-32.531, -80.0635) -> (-31.931, -79.0243)
  line L11 (-31.931, -79.0243) -> (-23.2707, -84.0243)
  line L12 (-15.1554, -91.25) -> (-16.2554, -93.1553)
  line L13 (-16.2554, -93.1553) -> (-5.8631, -99.1553)
  line L14 (-5.8631, -99.1553) -> (-4.7631, -97.25)
  line L15 (-4.7631, -97.25) -> (0, -100)
  line L16 (0, -100) -> (4.7631, -97.25)
  line L17 (4.7631, -97.25) -> (5.8631, -99.1553)
  line L18 (5.8631, -99.1553) -> (16.2554, -93.1553)
  line L19 (16.2554, -93.1553) -> (15.1554, -91.25)
  line L20 (15.1554, -91.25) -> (34.641, -80)
  line L21 (34.641, -80) -> (38.3731, -82.4641)
  line L22 (38.3731, -82.4641) -> (40.9711, -80.9641)
  line L23 (40.9711, -80.9641) -> (38.1051, -78)
  line L24 (38.1051, -78) -> (47.6314, -72.5)
  line L25 (47.6314, -72.5) -> (7.1252, -2.3412)
  arc A0 (4.7159, -5.8318) -> (7.1252, -2.3412) centre (0, 0) ccw
  line L26 (-37.2391, -78.5) -> (-15.1554, -91.25)
  line L27 (-6.4952, -95.0953) -> (-5.2452, -92.9302)
  line L28 (-5.2452, -92.9302) -> (-3.0801, -94.1802)
  line L29 (-3.0801, -94.1802) -> (-4.3301, -96.3453)
  line L30 (-4.3301, -96.3453) -> (-6.4952, -95.0953)
  line L31 (43.7993, -69.8627) -> (6.9282, -6)
  line L32 (6.9282, -6) -> (-33.407, -75.8627)
  line L33 (-33.407, -75.8627) -> (0, -95.1503)
  line L34 (0, -95.1503) -> (43.7993, -69.8627)
  line L35 (-37.2391, -78.5) -> (6.2697, -3.1406)
  dimension "d120" = 2
  dimension "d123" = 2
  dimension "d124" = 2
  dimension "d131" = 2
  constraint parallel L25 L31
  constraint parallel L26 L33
  constraint parallel L20 L34
  constraint coincident L26.start L35.start
  constraint parallel L32 L35
  measures "d120" distance of L25 L31
  measures "d123" distance of L11 L33
  measures "d124" distance of L7 L34
  measures "d131" distance of L32 L35
extrude "Extrude9" cut sketch "Sketch22" against normal blind 0.8 contours L31 L32 L33 L34
pattern_circular "C-Pattern7" count 6 over 360 about axis through (0, 0, 1.75) along (0, 0, 1) of "Extrude9"
sketch "Sketch23" plane through (0, 0, 12) normal (0.5, 0.866025, 0) x (0.866025, -0.5, 0)
  line L0 (115.8881, -20.3495) -> (-112.3469, -20.3495)
  line L1 (-112.3469, -20.3495) -> (-112.3469, 41.1723)
  line L2 (-112.3469, 41.1723) -> (115.8881, 41.1723)
  line L3 (115.8881, 41.1723) -> (115.8881, -20.3495)
  constraint horizontal L0
  constraint vertical L1
  constraint horizontal L2
  constraint vertical L3
ref_plane "WorkPlane5" through (51.7355, -74.3163, 3.6) normal (0, 0, 1) x (-1, 0, 0)
sketch "Sketch24" plane through (51.7355, -74.3163, 3.6) normal (0, 0, 1) x (1, 0, 0)
  line L0 (-10.7643, -6.6478, -0.6) -> (-10.7643, -6.6478, 3.4)
  line L1 (-14.9645, -9.0728) -> (-10.7643, -6.6478)
  line L2 (-10.7643, -6.6478) -> (-15.4645, -8.2068)
  line L3 (-15.4645, -8.2068) -> (-14.9645, -9.0728)
  line L4 (-10.7643, -6.6478, 3.4) -> (-13.3624, -8.1478, 3.4)
  point P0 (-10.7643, -6.6478)
  point P1 (-10.7643, -6.6478)
  point P2 (-13.3624, -8.1478)
  dimension "d134" = 90
  dimension "d135" = 4.85
  dimension "d136" = 1
  constraint coincident P0 L1.end
  constraint coincident P1 P0
  measures "d134" angle of L1 L3
  measures "d135" distance of L1.start P1
  measures "d136" distance of L1.start L2.end
extrude "Extrude10" cut sketch "Sketch24" along normal blind 3
pattern_circular "C-Pattern8" count 6 over 360 about axis through (0, 0, 1.75) along (0, 0, 1) of "Extrude10"
sketch "Sketch25" plane through (-87.1025, 0, 0) normal (1, 0, 0) x (0, 1, 0)
  line L0 (-5, 6.4) -> (-7, 6.4)
  line L1 (-7, 6.4) -> (-7, -0.4)
  line L2 (-7, -0.4) -> (-5, -0.4)
  line L3 (-5, -0.4) -> (-5, 6.4)
  line L4 (-7, 6.4) -> (-5, 6.4)
  line L5 (-5, 6.4) -> (-5, 3.4)
  line L6 (-5, 3.4) -> (-7, 3.4)
  line L7 (-7, 3.4) -> (-7, 6.4)
  dimension "d141" = 3
  constraint horizontal L4
  constraint vertical L5
  constraint horizontal L6
  constraint vertical L7
  constraint coincident L3 L5.end
  constraint coincident L0.end L1.start
  measures "d141" distance of L0.start L5.end
extrude "Extrude11" cut sketch "Sketch25" against normal blind 3.5 contours L0 L1 L3 L4 L5 L6 L7
pattern_circular "C-Pattern9" count 6 over 360 about axis through (0, 0, 1.75) along (0, 0, 1) of "Extrude11"
sketch "Sketch27" plane through (-43.3013, 75, 0) normal (0.5, -0.866025, 0) x (0.866025, 0.5, 0)
  line L0 (-32.5, 12) -> (-32.5, 0)
  line L1 (-32.5, 0) -> (-7, 0)
  line L2 (-7, 0) -> (-7, 6.4)
  line L3 (-7, 6.4) -> (-5, 6.4)
  line L4 (-5, 6.4) -> (-5, 0)
  line L5 (-5, 0) -> (6, 0)
  line L6 (6, 0) -> (6, 3)
  line L7 (6, 3) -> (10, 3)
  line L8 (10, 3) -> (10, 0)
  line L9 (10, 0) -> (32.5, 0)
  line L10 (32.5, 0) -> (32.5, 12)
  line L11 (32.5, 12) -> (-32.5, 12)
  line L12 (10, 7) -> (6, 7)
  line L13 (6, 7) -> (6, 10)
  line L14 (6, 10) -> (10, 10)
  line L15 (10, 10) -> (10, 7)
  line L16 (10, 10) -> (25, 10)
  line L17 (25, 10) -> (25, 7)
  line L18 (25, 7) -> (10, 7)
  line L19 (10, 7) -> (10, 10)
  line L20 (10, 3) -> (25, 3)
  line L21 (25, 3) -> (25, 0)
  line L22 (25, 0) -> (10, 0)
  line L23 (10, 0) -> (10, 3)
  line L24 (10, 10) -> (6, 10)
  line L25 (6, 10) -> (6, 7)
  line L26 (6, 7) -> (10, 7)
  line L27 (10, 7) -> (10, 10)
  line L28 (10, 3) -> (6, 3)
  line L29 (6, 3) -> (6, 0)
  line L30 (6, 0) -> (10, 0)
  line L31 (10, 0) -> (10, 3)
  line L32 (-7, 6.4) -> (-5, 6.4)
  line L33 (-5, 6.4) -> (-5, -0.4)
  line L34 (-5, -0.4) -> (-7, -0.4)
  line L35 (-7, -0.4) -> (-7, 6.4)
  line L36 (-5, -0.4, -0.5) -> (-5, -0.4, 81.0124)
  point P0 (-5, -0.4)
  point P1 (-5, -0.4)
  dimension "d146" = 15
  dimension "d147" = 15
  constraint horizontal L16
  constraint vertical L17
  constraint horizontal L18
  constraint vertical L19
  constraint coincident L14.end L15.start
  constraint horizontal L20
  constraint vertical L21
  constraint horizontal L22
  constraint vertical L23
  constraint coincident L9 L21.end
  constraint coincident L7.end L8.start
  constraint collinear L12 L18
  constraint horizontal L24
  constraint vertical L25
  constraint horizontal L26
  constraint vertical L27
  constraint coincident L12.end L13.start
  constraint horizontal L28
  constraint vertical L29
  constraint horizontal L30
  constraint vertical L31
  constraint coincident L5.end L6.start
  constraint horizontal L32
  constraint vertical L33
  constraint horizontal L34
  constraint vertical L35
  constraint coincident L2.end L3.start
  constraint collinear L4 L33
  constraint coincident P1 P0
  measures "d146" distance of L14.end L16.end
  measures "d147" distance of L7.end L20.end
extrude "Extrude12" cut sketch "Sketch27" against normal blind 2 contours L2 L3 L4 L32 L33 L34 L35 | L8 L9 L20 L21 L22 L23 L31 | L6 L7 L8 L23 L28 L29 L30 L31 | L12 L13 L14 L15 L19 L24 L25 L26 L27 | L15 L16 L17 L18 L19 L27
pattern_circular "C-Pattern10" count 6 over 360 about axis through (0, 0, 1.75) along (0, 0, 1) of "Extrude12"
equation "d9 = d10"
equation "d12 = 99.4226497308 mm / 3"
equation "d13 = ( 99.4226497308 mm / 3 ) * 2"
equation "d14 = d17"
equation "d15 = d17"
equation "d22 = d9 / 2"
equation "d23 = d9 / 2"
equation "d27 = d22 - d8"
equation "d29 = d27"
equation "d46 = d43"
equation "d47 = d41"
equation "d51 = d50"
equation "d60 = d59"
equation "d64 = d63"
equation "d85 = d84"
equation "d123 = d120"
equation "d124 = d120"
equation "d131 = d120"
equation "d147 = d146"
